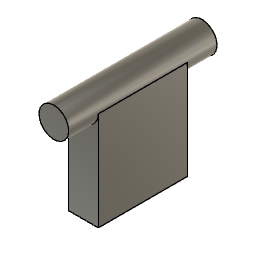
test1b v1 (Autodesk Fusion 360 design; units mm, degrees)
Autodesk Fusion 360 part; units mm, degrees
note: some values were not read from the file. Set by a fixed rule: which sketch regions a step uses.
sketch "Sketch1" plane through (0, 0, 0) normal (0, 1, 0) x (1, 0, 0)
  circle A0 centre (0, 0) radius 3
  line L0 (2.9999, 0.0269) -> (3, 0.0269)
  line L1 (3, 0.0269) -> (3, 20)
  line L2 (3, 20) -> (-3, 20)
  line L3 (-3, 20) -> (-3, 0)
  dimension "d1" = 6
  dimension "d2" = 6
  dimension "d3" = 20
  constraint coincident A0.centre origin
  constraint horizontal L0
  constraint vertical L1
  constraint horizontal L2
  constraint vertical L3
  constraint coincident A0 L3.end
  constraint coincident A0 L0.start
  constraint tangent A0 L1
  constraint tangent A0 L3
  measures "d1" diameter of A0
  measures "d2" distance of L1.end L2.end
  measures "d3" distance of A0.centre L2
extrude "Extrude1" add sketch "Sketch1" along normal mid plane 30 contours A0 makes body 1
extrude "Extrude2" add sketch "Sketch1" along normal mid plane 18 contours A0 L1 L2 L3 bodies 1
copy_body "Body->Comp1" bodies 1 removing the originals makes body 2 in component "Component"
component "Component" placed x (1, 0, 0) y (0, 1, 0) z (0, 0, 1) at (0, 0, 0)
